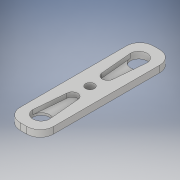
# Autodesk Inventor part: femur_v5
Saved by Autodesk Inventor 2019 (Build 230136000, 136)
## iProperties
Created: 2019-01-08
Part Number: femur_v5
Material: Generic
Document SubType Name: Modeling
Designer: Daniel
Density: 1 g/cm^3
Appearance: Default
Author: Daniel
Autodesk Inventor part; units mm, degrees
ref_plane "YZ Plane" through (0, 0, 0) normal (1, 0, 0) x (0, 1, 0)
ref_plane "XZ Plane" through (0, 0, 0) normal (0, 1, 0) x (-1, 0, 0)
ref_plane "XY Plane" through (0, 0, 0) normal (0, 0, 1) x (1, 0, 0)
sketch "Sketch1" plane through (0, 0, 0) normal (0, 1, 0) x (-1, 0, 0)
  line L0 (10.5, 0) -> (-10.5, 0) projected
  line L1 (0, -42) -> (0, 42) projected
  line L2 (7.5, -30) -> (-7.5, -30)
  line L3 (-7.5, -30) -> (-7.5, 30)
  line L4 (-7.5, 30) -> (7.5, 30)
  line L5 (7.5, 30) -> (7.5, -30)
  point P0 (0, 0)
  dimension "d0" = 15
  dimension "d1" = 60
  constraints: 8 end point, 2 parallel, 1 horizontal, 1 perpendicular, 2 other
  measures "d0" distance between parallel lines of L3 L5
  measures "d1" distance between parallel lines of L4 L2
extrude "Extrusion1" add sketch "Sketch1" along normal blind 3
sketch "Sketch2" plane through (0, 3, 0) normal (0, 1, 0) x (1, 0, 0)
  line L0 (7.5, 30) -> (-7.5, 30) projected
  line L1 (-7.5, 30) -> (-7.5, -30) projected
  line L2 (-7.5, -30) -> (7.5, -30) projected
  line L3 (7.5, -30) -> (7.5, 30) projected
  circle A0 centre (0, -22) radius 3.75
  circle A1 centre (0, -8) radius 2.5
  line L4 (0, 42) -> (0, -42) projected
  line L5 (-7.5, -5.5) -> (7.5, -5.5) construction
  line L6 (-2.4495, -7.5) -> (-3.75, -22)
  line L7 (3.75, -22) -> (2.4495, -7.5)
  line L8 (-10.5, 0) -> (10.5, 0) projected
  circle A2 centre (0, 22) radius 3.75
  circle A3 centre (0, 8) radius 2.5
  line L9 (-2.4495, 7.5) -> (-3.75, 22)
  line L10 (3.75, 22) -> (2.4495, 7.5)
  point P0 (0, 0)
  dimension "d4" = 7.5
  dimension "d5" = 8
  dimension "d6" = 5
  dimension "d9" = 16.5
  dimension "d10" = 2
  dimension "d11" = 8
  dimension "d12" = 8
  dimension "d13" = 2
  constraints: 10 end point, 8 point on circle, 6 symmetric about line, 4 centre point, 4 point on line, 1 horizontal, 1 tangent, 2 other
  measures "d4" diameter of A0
  measures "d5" distance from line of L2 A0.centre
  measures "d6" diameter of A1
  measures "d9" distance from line of A0.centre L5
  measures "d10" distance from line of L5 L7.end
  measures "d11" distance from line of L2 L7.start
  measures "d12" distance from line of L2 L6.end
  measures "d13" distance from line of L5 L6.start
extrude "Extrusion2" cut sketch "Sketch2" against normal blind 2 contours A2 L10 L4 | L4 A2 L9 | A2 L10 A3 L4 | L4 A3 L9 A2 | A3 L9 L4 | L4 A3 L10 | L4 A1 L6 | A1 L7 L4 | L4 A0 L7 | A0 L6 L4 | A1 L7 | L6 A1 | L4 A0 L6 A1 | A1 L7 A0 L4
sketch "Sketch3" plane through (0, 1, 0) normal (0, 1, 0) x (1, 0, 0)
  line L0 (7.5, 30) -> (-7.5, 30) projected
  line L1 (-7.5, 30) -> (-7.5, -30) projected
  line L2 (-7.5, -30) -> (7.5, -30) projected
  line L3 (7.5, -30) -> (7.5, 30) projected
  line L4 (-3.75, -22) -> (-2.4994, -8.0561) projected
  arc A0 (-3.75, -22) -> (3.75, -22) centre (0, -22) ccw projected
  line L5 (2.4994, -8.0561) -> (3.75, -22) projected
  arc A1 (2.4994, -8.0561) -> (-2.4994, -8.0561) centre (0, -8) ccw projected
  line L6 (3.75, 22) -> (2.4495, 7.5) projected
  arc A2 (3.75, 22) -> (-3.75, 22) centre (0, 22) ccw projected
  line L7 (-2.4495, 7.5) -> (-3.75, 22) projected
  arc A3 (-2.4495, 7.5) -> (2.4495, 7.5) centre (0, 8) ccw projected
  line L8 (-10.5, 0) -> (10.5, 0) projected
  point P0 (0, 0)
  constraints: 1 coincident, 1 symmetric about line
hole "Hole1" at (0, 1, 22) at (0, 1, -22) direction (0, -1, 0) diameter 7.5 end through all
fillet "Fillet1" radius 6 4 edges at (7.5, 1.5, -30) (-7.5, 1.5, -30) (-7.5, 1.5, 30) (7.5, 1.5, 30)
sketch "Sketch5" plane through (0, 3, 0) normal (0, 1, 0) x (1, 0, 0)
  arc A0 (3.75, 22) -> (-3.75, 22) centre (0, 22) ccw projected
  line L0 (3.75, 22) -> (2.4495, 7.5) projected
  arc A1 (-2.4495, 7.5) -> (2.4495, 7.5) centre (0, 8) ccw projected
  line L1 (-2.4495, 7.5) -> (-3.75, 22) projected
  line L2 (-3.75, -22) -> (-2.4994, -8.0561) projected
  arc A2 (2.4994, -8.0561) -> (-2.4994, -8.0561) centre (0, -8) ccw projected
  line L3 (2.4994, -8.0561) -> (3.75, -22) projected
  arc A3 (-3.75, -22) -> (3.75, -22) centre (0, -22) ccw projected
  arc A4 (1.5, -30) -> (7.5, -24) centre (1.5, -24) ccw projected
  line L4 (7.5, -24) -> (7.5, 24) projected
  arc A5 (7.5, 24) -> (1.5, 30) centre (1.5, 24) ccw projected
  line L5 (1.5, 30) -> (-1.5, 30) projected
  arc A6 (-1.5, 30) -> (-7.5, 24) centre (-1.5, 24) ccw projected
  line L6 (-7.5, 24) -> (-7.5, -24) projected
  arc A7 (-7.5, -24) -> (-1.5, -30) centre (-1.5, -24) ccw projected
  line L7 (-1.5, -30) -> (1.5, -30) projected
  point P0 (0, 0)
  point P1 (0, 0)
  constraints: 1 coincident
hole "Hole3" at (0, 3, 0) direction (0, -1, 0) diameter 4 end through all
body "Solid1"
